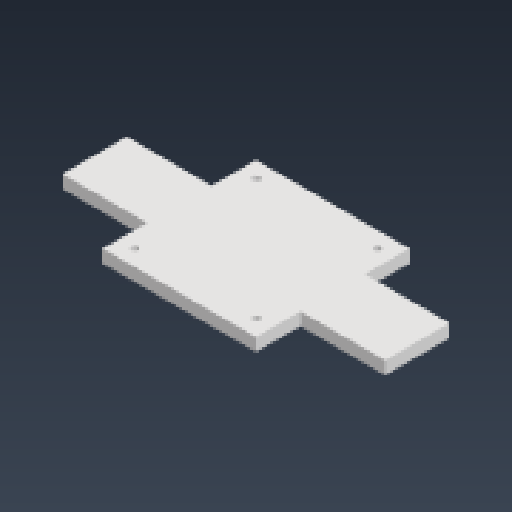
# Autodesk Inventor part: Power_box
Saved by Autodesk Inventor 2026.1 (Build 301233000, 233)
## iProperties
Created: 2026-02-06
Part Number: Power_box
Material: Generic
Document SubType Name: Modeling
Designer: aleja
Density: 1 g/cm^3
Appearance: Default
Author: aleja
Autodesk Inventor part; units mm, degrees
ref_plane "YZ Plane" through (0, 0, 0) normal (1, 0, 0) x (0, 1, 0)
ref_plane "XZ Plane" through (0, 0, 0) normal (0, 1, 0) x (-1, 0, 0)
ref_plane "XY Plane" through (0, 0, 0) normal (0, 0, 1) x (1, 0, 0)
sketch "Sketch1" plane through (0, 0, 0) normal (0, 0, 1) x (1, 0, 0)
  line L0 (-50, -50) -> (50, -50) construction
  line L1 (50, -50) -> (50, 50) construction
  line L2 (50, 50) -> (-50, 50) construction
  line L3 (-50, 50) -> (-50, -50) construction
  line L4 (-50, -50) -> (50, 50) construction
  line L5 (50, -50) -> (-50, 50) construction
  line L6 (-37.5, -37.5) -> (37.5, -37.5) construction
  line L7 (37.5, -37.5) -> (37.5, 37.5) construction
  line L8 (37.5, 37.5) -> (-37.5, 37.5) construction
  line L9 (-37.5, 37.5) -> (-37.5, -37.5) construction
  line L10 (-37.5, -37.5) -> (37.5, 37.5) construction
  line L11 (37.5, -37.5) -> (-37.5, 37.5) construction
  line L12 (-47.5, -47.5) -> (47.5, -47.5)
  line L13 (47.5, -47.5) -> (47.5, 47.5)
  line L14 (47.5, 47.5) -> (-47.5, 47.5)
  line L15 (-47.5, 47.5) -> (-47.5, -47.5)
  line L16 (-47.5, -47.5) -> (47.5, 47.5) construction
  line L17 (47.5, -47.5) -> (-47.5, 47.5) construction
  circle A0 centre (-50, 50) radius 2.15
  circle A1 centre (-37.5, 37.5) radius 2.15
  circle A2 centre (37.5, 37.5) radius 2.15
  circle A3 centre (-37.5, -37.5) radius 2.15
  circle A4 centre (37.5, -37.5) radius 2.15
  circle A5 centre (50, 50) radius 2.15
  circle A6 centre (-50, -50) radius 2.15
  circle A7 centre (50, -50) radius 2.15
  line L18 (-95, -20) -> (95, -20)
  line L19 (95, -20) -> (95, 20)
  line L20 (95, 20) -> (-95, 20)
  line L21 (-95, 20) -> (-95, -20)
  line L22 (-95, -20) -> (95, 20) construction
  line L23 (95, -20) -> (-95, 20) construction
  circle A8 centre (87.5, 0) radius 2.15
  line L24 (0, 0) -> (0, 12.464) construction
  circle A9 centre (-87.5, 0) radius 2.15
  point P0 (-47.5, -20)
  point P1 (-47.5, 20)
  point P2 (47.5, 20)
  point P3 (47.5, -20)
  dimension "d0" = 100
  dimension "d1" = 100
  dimension "d2" = 75
  dimension "d3" = 75
  dimension "d4" = 95
  dimension "d5" = 95
  dimension "d6" = 4.3
  dimension "d7" = 4.3
  dimension "d10" = 75
  dimension "d13" = 75
  dimension "d18" = 100
  dimension "d21" = 100
  dimension "d31" = 40
  dimension "d32" = 4.3
  dimension "d33" = 87.5
  dimension "d34" = 7.5
  constraints: 50 end point, 10 centre point, 8 midpoint, 8 parallel, 6 horizontal, 4 perpendicular, 3 coincident, 3 vertical, 1 symmetric about line, 13 other
  measures "d0" distance of L2.end L1.end
  measures "d1" distance of L1.end L0.end
  measures "d2" distance of L8.end L7.end
  measures "d3" distance of L7.end L6.end
  measures "d4" distance of L14.end L13.end
  measures "d5" distance of L13.end L12.end
  measures "d6" diameter of A0
  measures "d7" diameter of A1
  measures "d10" distance of A1.centre A2.centre
  measures "d13" distance of A1.centre A3.centre
  measures "d18" distance of A0.centre A5.centre
  measures "d21" distance of A0.centre A6.centre
  measures "d31" distance of L19.end L18.end
  measures "d32" diameter of A8
  measures "d33" distance of A8.centre point (0, 0)
  measures "d34" distance from line of L19 A8.centre
extrude "Extrusion1" add sketch "Sketch1" along normal blind 8 contours L15 L18 L13 L12 | L18 L21 L20 L15 | L15 L20 L13 L18 | L13 L20 L19 L18 | L15 L14 L13 L20
sketch "Sketch3" plane through (0, 0, 8) normal (0, 0, 1) x (1, 0, 0)
  line L0 (47.5, 47.5) -> (-47.5, 47.5) projected
  line L1 (-47.5, 47.5) -> (-47.5, 20) projected
  line L2 (-47.5, 20) -> (-95, 20) projected
  line L3 (-95, 20) -> (-95, -20) projected
  line L4 (-95, -20) -> (-47.5, -20) projected
  line L5 (-47.5, -20) -> (-47.5, -47.5) projected
  line L6 (-47.5, -47.5) -> (47.5, -47.5) projected
  line L7 (47.5, -47.5) -> (47.5, -20) projected
  line L8 (47.5, -20) -> (95, -20) projected
  line L9 (95, -20) -> (95, 20) projected
  line L10 (95, 20) -> (47.5, 20) projected
  line L11 (47.5, 20) -> (47.5, 47.5) projected
  line L12 (-27.5, -27.5) -> (27.5, -27.5)
  line L13 (27.5, -27.5) -> (27.5, 27.5)
  line L14 (27.5, 27.5) -> (-27.5, 27.5)
  line L15 (-27.5, 27.5) -> (-27.5, -27.5)
  line L16 (-27.5, -27.5) -> (27.5, 27.5) construction
  line L17 (27.5, -27.5) -> (-27.5, 27.5) construction
  line L18 (-65, -7.5) -> (65, -7.5)
  line L19 (65, -7.5) -> (65, 7.5)
  line L20 (65, 7.5) -> (-65, 7.5)
  line L21 (-65, 7.5) -> (-65, -7.5)
  line L22 (-65, -7.5) -> (65, 7.5) construction
  line L23 (65, -7.5) -> (-65, 7.5) construction
  point P0 (0, 0)
  point P1 (-27.5, 7.5)
  point P2 (-27.5, -7.5)
  point P3 (27.5, -7.5)
  point P4 (27.5, 7.5)
  dimension "d35" = 55
  dimension "d36" = 55
  dimension "d37" = 130
  dimension "d38" = 15
  constraints: 24 end point, 4 midpoint, 4 parallel, 2 horizontal, 2 perpendicular
  measures "d35" distance of L14.end L13.end
  measures "d36" distance of L13.end L12.end
  measures "d37" distance of L20.end L19.end
  measures "d38" distance of L19.end L18.end
extrude "Extrusion3" cut sketch "Sketch3" against normal through all contours L15 L18 L13 L12 | L18 L21 L20 L15 | L15 L20 L13 L18 | L13 L20 L19 L18 | L15 L14 L13 L20
fillet "Fillet1" radius 10 16 edges at (-47.5, -47.5, 4) (-47.5, -20, 4) (-95, -20, 4) (-47.5, 47.5, 4) (-95, 20, 4) (47.5, 47.5, 4) (95, 20, 4) (47.5, 20, 4) (95, -20, 4) (47.5, -20, 4) (47.5, -47.5, 4) (-47.5, 20, 4) (27.5, -7.5, 4) (27.5, 7.5, 4) (-27.5, 7.5, 4) (-27.5, -7.5, 4)
fillet "Fillet1" radius 5 6 edges at (27.5, 27.5, 4) (65, 7.5, 4) (65, -7.5, 4) (27.5, -27.5, 4) (-27.5, -27.5, 4) (-27.5, 27.5, 4)
equation "\"d1\" = d0"
equation "\"d5\" = d4"
equation "\"d35\" = d36"
body "Solid1"
